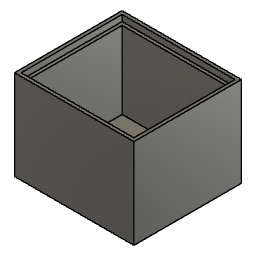
Stage_Cover (Autodesk Fusion 360 design; units mm, degrees)
Autodesk Fusion 360 part; units mm, degrees
sketch "base" plane through (0, 0, 0) normal (0, 1, 0) x (1, 0, 0)
  line L0 (36.5, -32.9) -> (-36.5, -32.9)
  line L1 (-36.5, -32.9) -> (-36.5, -30.9)
  line L2 (-36.5, -30.9) -> (36.5, -30.9)
  line L3 (36.5, -30.9) -> (36.5, -32.9)
  line L4 (36.5, 32.9) -> (-36.5, 32.9)
  line L5 (-36.5, 32.9) -> (-36.5, 30.9)
  line L6 (-36.5, 30.9) -> (36.5, 30.9)
  line L7 (36.5, 30.9) -> (36.5, 32.9)
  line L8 (36.5, -30.9) -> (34.5, -30.9)
  line L9 (34.5, -30.9) -> (34.5, 30.9)
  line L10 (34.5, 30.9) -> (36.5, 30.9)
  line L11 (36.5, 30.9) -> (36.5, -30.9)
  line L12 (0, -49.6148) -> (0, 45.2004) construction
  line L13 (54.9351, 0) -> (-34.717, 0) construction
  line L14 (-36.5, -30.9) -> (-34.5, -30.9)
  line L15 (-34.5, -30.9) -> (-34.5, 30.9)
  line L16 (-34.5, 30.9) -> (-36.5, 30.9)
  line L17 (-36.5, 30.9) -> (-36.5, -30.9)
  dimension "d1" = 2
  dimension "d2" = 73
  dimension "d3" = 65.8
  constraint horizontal L0
  constraint vertical L1
  constraint horizontal L2
  constraint vertical L3
  constraint horizontal L4
  constraint vertical L5
  constraint horizontal L6
  constraint vertical L7
  constraint equal L3 L7
  constraint equal L2 L6
  constraint collinear L3 L7
  constraint horizontal L8
  constraint vertical L9
  constraint horizontal L10
  constraint vertical L11
  constraint coincident L6 L9.end
  constraint equal L3 L8
  constraint vertical L12
  constraint horizontal L13
  constraint coincident origin L13
  constraint coincident origin L12
  constraint symmetric L2 L6 L13
  constraint symmetric L1 L3 L12
  constraint horizontal L14
  constraint vertical L15
  constraint horizontal L16
  constraint vertical L17
  constraint coincident L6 L15.end
  constraint equal L8 L14
  measures "d1" distance of L0.start L2.end
  measures "d2" distance of L0.start L0.end
  measures "d3" distance of L0 L4
extrude "Extrude1" add sketch "base" along normal blind 55 contours L0 L1 L2 L3 L8 L14 | L2 L6 L8 L9 L10 L11 | L2 L6 L14 L15 L16 L17 | L4 L5 L6 L7 L10 L16 makes body 1
extrude "Extrude2" add sketch "base" along normal blind 4 separate body contours L2 L6 L9 L15 makes body 2
sketch "Sketch3" plane through (0, 4, 0) normal (0, 1, 0) x (-1, 0, 0)
  line L0 (-34.5, 30.9) -> (-34.5, -30.9)
  line L1 (-34.5, -30.9) -> (34.5, -30.9)
  line L2 (34.5, -30.9) -> (34.5, 30.9)
  line L3 (34.5, 30.9) -> (-34.5, 30.9)
  line L4 (-32.5, -28.9) -> (32.5, -28.9)
  line L5 (32.5, -28.9) -> (32.5, 28.9)
  line L6 (32.5, 28.9) -> (-32.5, 28.9)
  line L7 (-32.5, 28.9) -> (-32.5, -28.9)
  dimension "d16" = -2
extrude "Extrude5" add sketch "Sketch3" along normal blind 47.2 bodies 1 2
equation "d17 = 56 mm - 3.8 mm - 5 mm"
